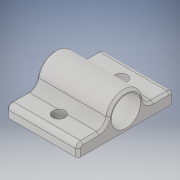
# Autodesk Inventor part: Prox_Z_3030
Saved by Autodesk Inventor 2019 (Build 230136000, 136)
## iProperties
Created: 2018-05-12
Part Number: Prox_Z_3030
Material: Generisch
Document SubType Name: Modeling
Designer: marc
Density: 1 g/cm^3
Appearance: Vorgabe
Author: marc
## iProperties of the stored document Prox_Z_3030_3D-Druck.ipt
Created: 2018-05-12
Part Number: Prox_Z_3030_3D-Druck
Material: Generisch
Document SubType Name: Modeling
Designer: marc
Density: 1 g/cm^3
Appearance: Vorgabe
Author: marc
Autodesk Inventor part; units mm, degrees
ref_plane "YZ Plane" through (0, 0, 0) normal (1, 0, 0) x (0, 1, 0)
ref_plane "XZ Plane" through (0, 0, 0) normal (0, 1, 0) x (-1, 0, 0)
ref_plane "XY Plane" through (0, 0, 0) normal (0, 0, 1) x (1, 0, 0)
sketch "Skizze1" plane through (0, 0, 0) normal (0, 1, 0) x (-1, 0, 0)
  line L0 (0, 0) -> (30, 0)
  line L1 (30, 0) -> (30, 40)
  line L2 (30, 40) -> (0, 40)
  line L3 (0, 40) -> (0, 0)
  circle A0 centre (15, 33) radius 2.55
  circle A1 centre (15, 7) radius 2.55
  dimension "d0" = 30
  dimension "d1" = 40
  dimension "d2" = 5.1
  dimension "d3" = 5.1
  dimension "d4" = 7
  dimension "d5" = 7
  dimension "d6" = 15
  dimension "d7" = 15
  constraints: 8 end point, 2 centre point, 2 parallel, 1 horizontal, 1 perpendicular
  measures "d0" distance of L2.end L1.end
  measures "d1" distance of L0.end L1.end
  measures "d2" diameter of A0
  measures "d3" diameter of A1
  measures "d4" distance from line of L2 A0.centre
  measures "d5" distance from line of L0 A1.centre
  measures "d6" distance from line of L3 A1.centre
  measures "d7" distance from line of A0.centre L3
extrude "Baseplate" add sketch "Skizze1" along normal blind 5
sketch "Skizze2" plane through (0, 0, 40) normal (1, 0, 0) x (0, 0, -1)
  arc A0 (27.2284, 5) -> (12.7716, 5) centre (20, 7) ccw
  line L0 (40, 0) -> (40, 5) projected
  line L1 (0, 5) -> (40, 5) projected
  line L2 (12.7716, 5) -> (27.2284, 5)
  line L3 (40, 5) -> (0, 5) projected
  dimension "d10" = 15
  dimension "d12" = 20
  dimension "d13" = 2
  constraints: 2 end point, 2 point on circle, 2 point on line, 1 centre point, 1 collinear
  measures "d10" diameter of A0
  measures "d12" distance from line of L0 A0.centre
  measures "d13" distance from line of L1 A0.centre
extrude "Rounding" add sketch "Skizze2" against normal up to surface (30 mm away)
sketch "Skizze3" plane through (0, 0, 40) normal (1, 0, 0) x (0, 0, -1)
  line L0 (40, 0) -> (40, 5) projected
  line L1 (27.2284, 5) -> (40, 5) projected
  circle A0 centre (20, 7) radius 4.05
  dimension "d17" = 20
  dimension "d18" = 2
  dimension "d19" = 8.1
  constraints: 1 centre point, 1 coincident
  measures "d17" distance from line of point (20, 7) L0
  measures "d18" distance from line of point (20, 7) L1
  measures "d19" diameter of A0
hole "Sensor" at (0, 7, 20) direction (-1, 0, 0) diameter 12.2 end through all
fillet "Rundung1" radius 4 2 edges at (-15, 5, 27.2284) (-15, 5, 12.7716)
fillet "Rundung2" radius 2 2 edges at (-15, 5, 0) (-15, 5, 40)
chamfer "Fase1" distance 1 angle 45 18 edges at (0, 1.5, 40) (0, 4.4142, 39.4142) (0, 5, 34.6624) (0, 5.9355, 28.754) (0, 5.9355, 11.246) (0, 14.5, 20) (0, 5, 5.3376) (0, 4.4142, 0.5858) (0, 1.5, 0) (-30, 5.9355, 28.754) (-30, 5.9355, 11.246) (-30, 14.5, 20) (-30, 5, 34.6624) (-30, 4.4142, 39.4142) (-30, 1.5, 40) (-30, 5, 5.3376) (-30, 4.4142, 0.5858) (-30, 1.5, 0)
equation "\"d3\" = d2"
equation "\"d5\" = d4"
